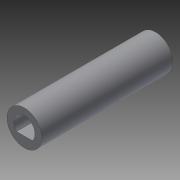
# Autodesk Inventor part: ShaftConverter
Saved by Autodesk Inventor 2013 (Build 170138000, 138)
## iProperties
Created: 2013-11-09
Part Number: ShaftConverter
Material: Generic
Document SubType Name: Modeling
Designer: JustinIndra
Density: 1 g/cm^3
Author: JustinIndra
Autodesk Inventor part; units mm, degrees
ref_plane "YZ Plane" through (0, 0, 0) normal (1, 0, 0) x (0, 1, 0)
ref_plane "XZ Plane" through (0, 0, 0) normal (0, 1, 0) x (-1, 0, 0)
sketch "Sketch1" plane through (0, 0, 0) normal (0, 1, 0) x (-1, 0, 0)
  circle A0 centre (0, 0) radius 1.5
  circle A1 centre (0, 0) radius 2.45
  line L0 (1.118, -1) -> (-1.118, -1)
  line L1 (0.4634, -1.5) -> (-1.27, -1.5) construction
  arc A2 (-1.118, -1) -> (1.118, -1) centre (0, 0) ccw construction
  dimension "d0" = 3
  dimension "d1" = 4.9
  dimension "d2" = 0.5
  constraints: 4 end point, 4 point on circle, 3 centre point, 2 coincident, 1 horizontal, 1 parallel, 1 tangent
  measures "d0" diameter of A0
  measures "d1" diameter of A1
  measures "d2" distance between parallel lines of L0 L1
extrude "Extrusion1" add sketch "Sketch1" along normal mid plane 18.5 contours L0 A0 | A1 picked at (-0.2826, -1.0791)
ref_plane "Work Plane1" through (0, 0, -2.45) normal (0, 0, 1) x (1, 0, 0)
sketch "Sketch6" plane through (0, 0, -2.45) normal (0, 0, 1) x (1, 0, 0)
  line L0 (2.5, 5.25) -> (-2.5, 5.25)
  line L1 (-2.5, 5.25) -> (-2.5, -0.75)
  line L2 (-2.5, -0.75) -> (2.5, -0.75)
  line L3 (2.5, -0.75) -> (2.5, 5.25)
  line L4 (2.45, 9.25) -> (-2.45, 9.25) projected
  point P0 (0, 0)
  point P1 (0, 5.25)
  dimension "d20" = 4
  dimension "d21" = 6
  dimension "d22" = 5
  constraints: 8 end point, 2 parallel, 1 horizontal, 1 midpoint, 1 perpendicular, 1 vertical alignment
  measures "d20" distance between parallel lines of L4 L0
  measures "d21" distance of L0.end L1.end
  measures "d22" distance of L1.end L2.end
extrude "Extrusion6" cut sketch "Sketch6" along normal blind 0.5
body "Solid1"
